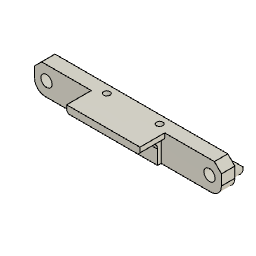
AfterburnerADXLMount (Autodesk Fusion 360 design; units mm, degrees)
Autodesk Fusion 360 part; units mm, degrees
sketch "Sketch1" plane through (0, 0, 0) normal (0, 1, 0) x (1, 0, 0)
  line L0 (26.5, -4) -> (-26.5, -4)
  line L1 (-26.5, -4) -> (-26.5, 4)
  line L2 (-26.5, 4) -> (26.5, 4)
  line L3 (26.5, 4) -> (26.5, -4)
  line L4 (26.5, -4) -> (-26.5, 4) construction
  line L5 (-26.5, -4) -> (26.5, 4) construction
  circle A0 centre (-23.109, 0) radius 1.6
  circle A1 centre (23.109, 0) radius 1.6
  line L6 (-23.109, 0) -> (0, 0) construction
  line L7 (0, 0) -> (23.109, 0) construction
  dimension "d1" = 46.218
  dimension "d2" = 3.2
  dimension "d3" = 53
  dimension "d4" = 8
  constraint horizontal L0
  constraint perpendicular L0 L1
  constraint parallel L0 L2
  constraint parallel L1 L3
  constraint coincident L4 L6.end
  constraint coincident L5 L6.end
  constraint coincident L6.end L7.start
  constraint coincident A0.centre L6.start
  constraint horizontal L6
  constraint coincident A1.centre L7.end
  constraint parallel L6 L7
  constraint equal L6 L7
  constraint equal A0 A1
  measures "d1" distance of A0.centre A1.centre
  measures "d2" diameter of A0
  measures "d3" distance of L1.end L2.end
  measures "d4" distance of L0.start L2.end
extrude "Extrude1" add sketch "Sketch1" along normal blind 13.8
sketch "Sketch3" plane through (0, 0, 4) normal (0, 0, 1) x (-1, 0, 0)
  line L0 (26.5, 0) -> (-26.5, 0)
  line L1 (-26.5, 0) -> (-26.5, -13.8)
  line L2 (-26.5, -13.8) -> (26.5, -13.8)
  line L3 (26.5, -13.8) -> (26.5, 0)
  line L4 (0, 0) -> (0, -13.8) construction
  line L5 (0, -11.5) -> (-7.5, -11.5) construction
  line L6 (0, -11.5) -> (7.5, -11.5) construction
  circle A0 centre (7.5, -11.5) radius 0.9
  circle A1 centre (-7.5, -11.5) radius 0.9
  dimension "d7" = 15
  dimension "d8" = 1.8
  dimension "d9" = 2.3
  constraint coincident L4.start origin
  constraint midpoint L2 L4.end
  constraint coincident L4 L5.start
  constraint perpendicular L4 L5
  constraint perpendicular L4 L6
  constraint equal L5 L6
  constraint coincident L6.end A0.centre
  constraint coincident L5.end A1.centre
  constraint equal A0 A1
  measures "d7" distance of L5.end L6.end
  measures "d8" diameter of A0
  measures "d9" distance of L2 L6
extrude "Extrude2" cut sketch "Sketch3" against normal through all contours A0 | A1
sketch "Sketch5" plane through (0, 13.8, 0) normal (0, 1, 0) x (-1, 0, 0)
  circle A0 centre (-23.109, 0) radius 1.6
  circle A1 centre (23.109, 0) radius 1.6
  line L0 (-26.5, -4) -> (26.5, -4)
  line L1 (26.5, -4) -> (26.5, 4)
  line L2 (26.5, 4) -> (-26.5, 4)
  line L3 (-26.5, 4) -> (-26.5, -4)
  circle A2 centre (-23.109, 0) radius 2.95
  circle A3 centre (23.109, 0) radius 2.95
  dimension "d11" = 5.9
  constraint concentric A0 A2
  constraint concentric A1 A3
  constraint equal A2 A3
  measures "d11" diameter of A3
extrude "Extrude3" add sketch "Sketch5" along normal blind 3.2 contours A2 | A3
fillet "Fillet1" radius 0.4 2 edges at (25.8594, 17, -1.0668) (-20.3586, 17, -1.0668)
extrude "Extrude4" cut 1 faces at (7.4363, 0, -3.1285) along direction (0, 1, 0) blind 10
sketch "Sketch7" plane through (0, 10, 0) normal (0, -1, 0) x (1, 0, 0)
  circle A0 centre (23.109, 0) radius 1.6
  circle A1 centre (-23.109, 0) radius 1.6
  line L0 (-26.5, -4) -> (26.5, -4)
  line L1 (26.5, -4) -> (26.5, 4)
  line L2 (26.5, 4) -> (-26.5, 4)
  line L3 (-26.5, 4) -> (-26.5, -4)
  circle A2 centre (-23.109, 0) radius 3
  circle A3 centre (23.109, 0) radius 3
  line L4 (-10.4, 4) -> (10.4, 4)
  line L5 (10.4, 4) -> (10.4, 2)
  line L6 (10.4, 2) -> (-10.4, 2)
  line L7 (-10.4, 2) -> (-10.4, 4)
  line L8 (-8.4, 4) -> (-6.6, 4)
  line L9 (6.6, 4) -> (8.4, 4)
  line L10 (-9.4, 2) -> (9.4, 2)
  line L11 (9.4, 2) -> (9.4, -4)
  line L12 (9.4, -4) -> (-9.4, -4)
  line L13 (-9.4, -4) -> (-9.4, 2)
  dimension "d20" = 6
  dimension "d21" = 6
  dimension "d22" = 2
  dimension "d23" = 2
  dimension "d24" = 2
  dimension "d25" = 1
  dimension "d26" = 1
  constraint concentric A1 A2
  constraint concentric A0 A3
  constraint horizontal L4
  constraint vertical L5
  constraint horizontal L6
  constraint vertical L7
  constraint coincident L2 L4.start
  constraint horizontal L10
  constraint vertical L11
  constraint horizontal L12
  constraint vertical L13
  constraint coincident L0 L11.end
  constraint coincident L6 L10.start
  measures "d20" diameter of A2
  measures "d21" diameter of A3
  measures "d22" distance of L4.start L8.start
  measures "d23" distance of L4.end L9.end
  measures "d24" distance of L4.end L5.end
  measures "d25" horizontal distance of L8.start L10.start
  measures "d26" horizontal distance of L9.end L10.end
extrude "Extrude5" add sketch "Sketch7" along normal blind 1 contours L0 L6 L10 L11 L12 L13 | L2 L4 L5 L6 L7 L8 L9 L10
sketch "Sketch8" plane through (0, 9, 0) normal (0, -1, 0) x (1, 0, 0)
  line L0 (-9.4, -4) -> (9.4, -4)
  line L1 (9.4, -4) -> (9.4, 2)
  line L2 (9.4, 2) -> (10.4, 2)
  line L3 (10.4, 2) -> (10.4, 4)
  line L4 (10.4, 4) -> (-10.4, 4)
  line L5 (-10.4, 4) -> (-10.4, 2)
  line L6 (-10.4, 2) -> (-9.4, 2)
  line L7 (-9.4, 2) -> (-9.4, -4)
  line L8 (-10.4, 4) -> (10.4, 4)
  line L9 (10.4, 4) -> (10.4, 2)
  line L10 (10.4, 2) -> (-10.4, 2)
  line L11 (-10.4, 2) -> (-10.4, 4)
  constraint horizontal L8
  constraint vertical L9
  constraint horizontal L10
  constraint vertical L11
  constraint coincident L2.end L3.start
  constraint coincident L4.end L5.start
extrude "Extrude6" add sketch "Sketch8" along normal blind 6 contours L2 L3 L4 L5 L6 L8 L9 L10 L11
fillet "Fillet3" radius 2 1 edges at (0, 9, 2)
fillet "Fillet4" radius 3 2 edges at (26.5, 11.9, -4) (-26.5, 11.9, -4)
chamfer "Chamfer1" distance 2 angle 45 2 edges at (-26.5, 11.9, 4) (26.5, 11.9, 4)
sketch "Sketch9" plane through (-26.5, 0, 0) normal (-1, 0, 0) x (0, -1, 0)
  line L0 (-10, 2) -> (-13.8, 2)
  line L1 (-13.8, 2) -> (-13.8, -1)
  line L2 (-13.8, -1) -> (-10, -1)
  line L3 (-10, -1) -> (-10, 2)
  line L4 (-13.8, -2.95) -> (-13.8, 2.95)
  line L5 (-16.6, 2.95) -> (-16.6, -2.95) construction
  line L6 (-17, -2.55) -> (-17, 2.55)
  line L7 (-13.8, 2.95) -> (-17, -0.25)
  line L8 (-13.8, 2.95) -> (-17, 2.95)
  line L9 (-17, -0.25) -> (-17, 2.95)
  dimension "d36" = 45
  constraint coincident L4.end L7.start
  constraint coincident L6 L7.end
  constraint perpendicular L4 L8
  constraint coincident L8 L9.end
  constraint perpendicular L8 L9
  measures "d36" angle of L4 L7
extrude "Extrude7" cut sketch "Sketch9" against normal through all contours L6 L7 L8 L9
chamfer "Chamfer2" distance 0.6 angle 45 2 edges at (-10.4, 6.5, 2) (10.4, 6.5, 2)
